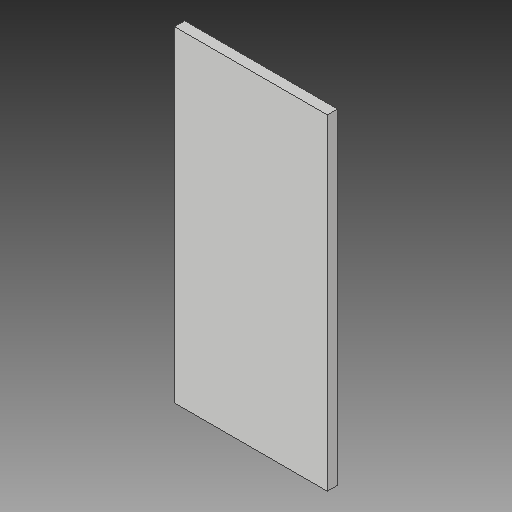
# Autodesk Inventor part: Placa
Saved by Autodesk Inventor 2017 (Build 210142000, 142)
## iProperties
Part Number: Placa
Material: Genérico
Document SubType Name: Modeling
Designer: osvaldo
Density: 1 g/cm^3
Appearance: Valor por defecto
Author: osvaldo
Autodesk Inventor part; units mm, degrees
ref_plane "YZ Plane" through (0, 0, 0) normal (1, 0, 0) x (0, 1, 0)
ref_plane "XZ Plane" through (0, 0, 0) normal (0, 1, 0) x (-1, 0, 0)
ref_plane "XY Plane" through (0, 0, 0) normal (0, 0, 1) x (1, 0, 0)
sketch "Boceto1" plane through (0, 0, 0) normal (0, 0, 1) x (1, 0, 0)
  line L0 (37.5, -80) -> (-37.5, -80)
  line L1 (-37.5, -80) -> (-37.5, 80)
  line L2 (-37.5, 80) -> (37.5, 80)
  line L3 (37.5, 80) -> (37.5, -80)
  line L4 (37.5, -80) -> (-37.5, 80) construction
  line L5 (-37.5, -80) -> (37.5, 80) construction
  point P0 (0, 0)
  dimension "d0" = 160
  dimension "d1" = 75
  constraints: 12 end point, 2 midpoint, 2 parallel, 1 horizontal, 1 perpendicular
  measures "d0" distance of L0.end L1.end
  measures "d1" distance of L1.end L2.end
extrude "Extrusión1" add sketch "Boceto1" against normal blind 5
equation "\"d0\" = 160 * scale"
equation "\"d1\" = 75 * scale"
equation "\"d2\" = 5 * scale"
equation "\"scale\" = 1"
